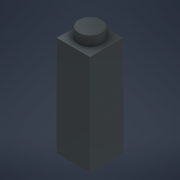
# Autodesk Inventor part: 110033226_ipt_24_直條(3x1)
Saved by Autodesk Inventor 2022 (Build 260153000, 153)
## iProperties
Created: 2022-06-23
Part Number: 110033226_ipt_24_直條(3x1)
Material: 一般
Document SubType Name: Modeling
Designer: User
Density: 1 g/cm^3
Appearance: 預設
Author: User
Autodesk Inventor part; units mm, degrees
ref_plane "YZ Plane" through (0, 0, 0) normal (1, 0, 0) x (0, 1, 0)
ref_plane "XZ Plane" through (0, 0, 0) normal (0, 1, 0) x (-1, 0, 0)
ref_plane "XY Plane" through (0, 0, 0) normal (0, 0, 1) x (1, 0, 0)
sketch "草圖1" plane through (0, 0, 0) normal (0, 1, 0) x (-1, 0, 0)
  line L0 (5, 0) -> (0, 0)
  line L1 (0, 0) -> (0, -5)
  line L2 (0, -5) -> (5, -5)
  line L3 (5, -5) -> (5, 0)
  circle A0 centre (2.5, -2.5) radius 1.7
  point P0 (2.5, -5)
  point P1 (5, -2.5)
  dimension "d0" = 5
  dimension "d1" = 5
  dimension "d2" = 3.4
  constraints: 8 end point, 2 midpoint, 2 parallel, 1 centre point, 1 coincident, 1 horizontal, 1 horizontal alignment, 1 perpendicular, 1 vertical alignment
  measures "d0" distance of L2.end L1.end
  measures "d1" distance of L1.end L0.end
  measures "d2" diameter of A0
extrude "擠出1" add sketch "草圖1" along normal blind 15 contours L3 L2 L1 L0 | A0
extrude "擠出2" cut sketch "草圖1" along normal blind 1.5 contours A0
sketch "草圖2" plane through (0, 15, 0) normal (0, 1, 0) x (1, 0, 0)
  circle A0 centre (-2.5, 2.5) radius 1.7 projected
  point P0 (0, 0)
extrude "擠出3" add sketch "草圖2" along normal blind 1.5
sketch "草圖3" plane through (0, 0, 0) normal (1, 0, 0) x (0, 1, 0)
  line L0 (8.7779, 7.7621) -> (6.2221, 7.7621)
  line L1 (6.2221, 7.7621) -> (6.2221, -14.483)
  line L2 (6.2221, -14.483) -> (8.7779, -14.483)
  line L3 (8.7779, -14.483) -> (8.7779, 7.7621)
  line L4 (0, -5) -> (15, -5) projected
  point P0 (0, 0)
  point P1 (7.5, -14.483)
  point P2 (7.5, -5)
  constraints: 8 end point, 2 midpoint, 2 parallel, 1 horizontal, 1 perpendicular, 1 vertical alignment
split_face "分割1"
